Autodesk Fusion 360 part; units mm, degrees
(part 2 of 2)
sketch "Sketch1 (2)" plane through (5.45, -12.4, 0) normal (0, 1, 0) x (-1, 0, 0) in component "ServoTrayMount"
  line L0 (-16.2, -6.2) -> (-11.2, -6.2) construction
  line L1 (-16.2, 6.2) -> (-16.2, -6.2) construction
  line L2 (-16.2, -0.6) -> (-15.053256, -0.6) construction
  line L3 (-16.2, 0.6) -> (-15.053256, 0.6) construction
  circle A0 centre (-13.9, 0) radius 1.3
  line L4 (-11.2, 6.2) -> (-16.2, 6.2) construction
  line L5 (-11.2, 0) -> (-11.2, 12.4) construction
  line L6 (-11.2, 0) -> (-11.2, -12.4) construction
  line L7 (11.2, -6.2) -> (11.2, 0) construction
  line L8 (16.2, -6.2) -> (11.2, -6.2) construction
  line L9 (16.2, 6.2) -> (16.2, -6.2) construction
  line L10 (16.2, 0.6) -> (15.053256, 0.6) construction
  line L11 (16.2, -0.6) -> (15.053256, -0.6) construction
  circle A1 centre (13.9, 0) radius 1.3
  line L12 (11.2, 6.2) -> (11.2, 0) construction
  line L13 (11.2, 6.2) -> (16.2, 6.2) construction
  line L14 (-11.2, 6.2) -> (11.2, 6.2) construction
  line L15 (-11.2, -6.2) -> (11.2, -6.2) construction
  circle A2 centre (5.45, 0) radius 1
  line L16 (-16.2, -6.2) -> (-16.2, -6.4) construction
  line L17 (-16.2, -6.4) -> (-16.4, -6.4) construction
  line L18 (16.2, 6.2) -> (16.2, 6.4) construction
  line L19 (16.2, 6.4) -> (16.4, 6.4) construction
  line L20 (16.4, 6.4) -> (-16.4, 6.4)
  line L21 (-16.4, 6.4) -> (-16.4, -6.4)
  line L22 (-16.4, -6.4) -> (16.4, -6.4)
  line L23 (16.4, -6.4) -> (16.4, 6.4)
  line L24 (-16.4, -6.4) -> (-16.4, -9.4) construction
  line L25 (-11.2, -6.4) -> (-11.4, -6.4)
  line L26 (-11.4, -6.4) -> (-11.4, 6.4)
  line L27 (0, -6.2) -> (0, 6.2) construction
  line L28 (11.4, -6.4) -> (11.4, 6.4)
  line L29 (-16.4, -9.4) -> (-15.4, -9.4)
  line L30 (-15.4, -9.4) -> (-16.2, -9.4)
  line L31 (15.4, -9.4) -> (16.2, -9.4)
  line L32 (-16.2, 0) -> (16.2, 0) construction
  line L33 (15.4, 9.4) -> (16.2, 9.4)
  line L34 (16.2, 9.4) -> (-16.2, 9.4)
  line L35 (-16.2, 9.4) -> (-16.2, -9.4)
  line L36 (-16.2, -9.4) -> (16.2, -9.4)
  line L37 (16.2, -9.4) -> (16.2, 9.4)
  dimension "TrayGap" = 0.2
  dimension "d123" = 0.2
  dimension "d124" = 0.2
  dimension "d125" = 0.2
  dimension "TraySideWidth" = 3
  dimension "d127" = 0.2
  dimension "d128" = 1
  dimension "TrayEndExtraMinus1" = 0.8
  constraint coincident L0.start L1.end
  constraint vertical L16
  constraint perpendicular L16 L17
  constraint coincident L9.start L13.end
  constraint perpendicular L13 L18
  constraint perpendicular L18 L19
  constraint horizontal L20
  constraint vertical L21
  constraint horizontal L22
  constraint vertical L23
  constraint perpendicular L17 L24
  constraint coincident L6 L25.start
  constraint coincident L22 L25.start
  constraint perpendicular L6 L25
  constraint coincident L20 L26.end
  constraint perpendicular L20 L26
  constraint midpoint L15 L27.start
  constraint midpoint L14 L27.end
  constraint symmetric L25.end L27 L28.start
  constraint symmetric L26.end L27 L28.end
  constraint perpendicular L24 L29
  constraint parallel L29 L30
  constraint symmetric L27 L29.end L31.start
  constraint symmetric L27 L30.end L31.end
  constraint midpoint L1 L32.start
  constraint midpoint L9 L32.end
  constraint symmetric L31.start L32 L33.start
  constraint symmetric L31.end L32 L33.end
  constraint horizontal L34
  constraint vertical L35
  constraint horizontal L36
  constraint vertical L37
  measures "TrayGap" distance of L0.start L16.end
  measures "d123" distance of L16.end L17.end
  measures "d124" distance of L9.start L18.end
  measures "d125" distance of L18.end L19.end
  measures "TraySideWidth" distance of L17.end L24.end
  measures "d127" distance of L25.start L25.end
  measures "d128" distance of L24.end L29.end
  measures "TrayEndExtraMinus1" distance of L29.end L30.end
extrude "Extrude1''" add sketch "Sketch1 (2)" along normal blind 3 separate body contours L20 L33 L34 L35 L37 | L20 L22 L28 L37 | L20 L22 L26 L35 | L22 L25 L29 L30 L31 L35 L36 L37 picked at (-4.066667, 8.4) picked at (13.80095, -4.698788) picked at (-13.80095, 4.698788) picked at (-3.733333, -8.4) makes body 10 in component "ServoTrayMount"
component "Servo" placed x (1, 0, 0) y (0, 1, 0) z (0, 0, 1) at (0, 0, 0)
component "Shaft" placed x (1, 0, 0) y (0, 1, 0) z (0, 0, 1) at (0, 0, 0) in component "Servo"
component "Horn" placed x (1, 0, 0) y (0, 1, 0) z (0, 0, 1) at (0, 0, 0) in component "Servo"
component "Joint" placed x (1, 0, 0) y (0, 1, 0) z (0, 0, 1) at (0, 0, 0) in component "Servo"
component "ServoTrayMount" placed x (1, 0, 0) y (0, 1, 0) z (0, 0, 1) at (0, 0, 0) in component "Servo"
hidden bodies 2
equation "NumSplines = 20"
equation "d7 = ShaftOuterDia / 4"
equation "SplineTipPointiness = ShaftOuterDia * PI / NumSplines / 8"
equation "SplineInnerPointiness = ShaftOuterDia * PI / NumSplines / 8"
equation "ShaftHeight = 3.5 mm"
equation "d13 = ScrewholeDia + 0.5 * ( ( ShaftSplinesInnerDia - ScrewholeDia ) )"
equation "d20 = -ShaftHeight"
equation "d22 = -ShaftHeight"
equation "d24 = NumSplines"
equation "d26 = ScrewholeDia"
equation "ShaftScrewSectionsize = 0.2 mm"
equation "ShaftScrewPitch = ShaftHeight / 0.4 mm"
equation "d30 = -ShaftHeight"
equation "d31 = -ShaftHeight"
equation "n = 14.5 mm"
equation "d36 = HatTipDia / 2"
equation "HatHeight = 4.5 mm"
equation "Hole_to_closest_end_dist = HatDia / 2"
equation "ServoBodyHeight = 24 mm"
equation "ServoCornerWireRecess = 3 mm"
equation "ServoTabRecess = -4.4 mm"
equation "d47 = ServoBodyWidth"
equation "d48 = ServoTabSize"
equation "d49 = ServoBodyWidth"
equation "d52 = TabScrewSize / 2"
equation "d53 = ServoBodyWidth / 2"
equation "d55 = ( ServoBodyWidth - TabScrewGapSize ) / 2"
equation "TabThickness = -2.4 mm"
equation "d61 = WireHoleHeight"
equation "d62 = WireHoleWidth / 2"
equation "d63 = WireHoleWidth"
equation "d64 = WireHoleHeight"
equation "d65 = WireHoleWidth / 4"
equation "d66 = WireHoleWidth / 4 + 0.1 mm"
equation "d67 = WireHoleWidth / 4"
equation "d68 = -WireHoleWidth"
equation "WireLenght = 5 mm"
equation "OuterHubDia = 7.3 mm + 2 * tol"
equation "MajorArmLen = 36.2 mm + 2 * tol"
equation "MinroArmLen = 19 mm + 2 * tol"
equation "TipDiaMajor = 5 mm + 2 * tol"
equation "TipDiaMinor = 4 mm + 2 * tol"
equation "d14 = DriveHole"
equation "d19 = OuterHubDia + 1.5 mm + tol + 2 * tol"
equation "d90 = OuterHubDia + 2 * tol"
equation "ReinforcerWidth = 1 mm + 2 * tol"
equation "d92 = ReinforcerWidth / 2 + tol"
equation "HornCollarDepth = -2.7 mm"
equation "HornUnderside = -1 mm"
equation "HornInnerScrewTabThickness = 1.2 mm"
equation "HornUpperHeight = 2.3 mm"
equation "d103 = HornUpperHeight / 3"
equation "HornArmTopSide = -1.5 mm"
equation "d123 = TrayGap"
equation "d124 = TrayGap"
equation "d125 = TrayGap"
equation "d127 = TrayGap"
equation "TrayEndExtraMinus1 = 1 mm - TrayGap"
equation "ServoTrayThickness = 3 mm"
named bodies: "Ignore", "Shaft", "Thread", "ServoBody", "Signal", "Positive", "Ground", "ServoHorn", "ServoTrayMount"
